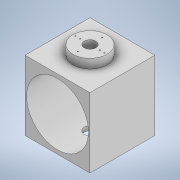
# Autodesk Inventor part: engine_connector_sleeve
Saved by Autodesk Inventor 2020.1 (Build 241239000, 239)
## iProperties
Created: 2022-02-06
Part Number: engine_connector_sleeve
Material: Generic
Document SubType Name: Modeling
Designer: OEM
Density: 1 g/cm^3
Appearance: Default
Author: OEM
Autodesk Inventor part; units mm, degrees
ref_plane "YZ Plane" through (0, 0, 0) normal (1, 0, 0) x (0, 1, 0)
ref_plane "XZ Plane" through (0, 0, 0) normal (0, 1, 0) x (-1, 0, 0)
ref_plane "XY Plane" through (0, 0, 0) normal (0, 0, 1) x (1, 0, 0)
sketch "Sketch1" plane through (0, 0, 0) normal (0, 1, 0) x (-1, 0, 0)
  circle A0 centre (0, 0) radius 11
  circle A1 centre (0, 0) radius 3
  circle A2 centre (0, 0) radius 3.75
  circle A3 centre (0, 0) radius 6.375 construction
  circle A4 centre (0, 0) radius 9.375 construction
  circle A5 centre (0, 0) radius 7.875 construction
  circle A6 centre (0, -7.875) radius 0.35
  circle A7 centre (6.375, 0) radius 0.35
  circle A8 centre (9.375, 0) radius 0.35
  line L0 (16.292, 0) -> (-19, 0) construction
  line L1 (0, 21) -> (0, -27.3544) construction
  circle A9 centre (0, 7.875) radius 0.35
  circle A10 centre (-6.375, 0) radius 0.35
  circle A11 centre (-9.375, 0) radius 0.35
  line L2 (0, -21) -> (21, -21)
  line L3 (21, -21) -> (21, 0)
  line L4 (0, 21) -> (21, 21)
  line L5 (21, 21) -> (21, 0)
  line L6 (0, -21) -> (-21, -21)
  line L7 (-21, -21) -> (-21, 0)
  line L8 (-21, 21) -> (-21, 0)
  line L9 (0, 21) -> (-21, 21)
  dimension "d6" = 12.75
  dimension "d7" = 18.75
  dimension "d8" = 15.75
  dimension "d2" = 7.5
  dimension "d4" = 22
  dimension "d5" = 6
  dimension "d9" = 0.7
  dimension "d13" = 0.7
  dimension "d14" = 0.7
  dimension "d17" = 21
  dimension "d18" = 21
  constraints: 20 end point, 9 centre point, 7 symmetric about line, 6 coincident, 2 horizontal alignment, 1 horizontal, 1 perpendicular, 1 point on line, 1 vertical, 1 vertical alignment, 9 other
  measures "d2" diameter of A2
  measures "d4" diameter of A0
  measures "d5" diameter of A1
  measures "d9" diameter of A6
  measures "d13" diameter of A7
  measures "d14" diameter of A8
  measures "d17" distance from line of point (0, 0) L2
  measures "d18" distance from line of A0.centre L3
extrude "Extrusion1" add sketch "Sketch1" against normal blind 45 contours A0 | A6 | A7 | A8 | A9 | A10 | A11 | L6 L7 L8 L9 L4 L5 L3 L2
extrude "Extrusion2" add sketch "Sketch1" along normal blind 6 contours A0
sketch "Sketch2" plane through (-21, 0, 21) normal (0, 0, 1) x (1, 0, 0)
  line L0 (42, 0) -> (0, 0) construction
  line L1 (42, 0) -> (42, -45) construction
  line L2 (42, -45) -> (0, -45) construction
  line L3 (0, 0) -> (0, -45) construction
  line L4 (42, -45) -> (0, -45) construction
  line L5 (0, 0) -> (0, -45) construction
  line L6 (42, 0) -> (0, -45) construction
  line L7 (42, -45) -> (0, 0) construction
  circle A0 centre (21, -22.5) radius 20
  point P0 (21, 0)
  dimension "d23" = 40
  constraints: 8 end point, 2 perpendicular, 1 centre point, 1 midpoint
  measures "d23" diameter of A0
extrude "Extrusion3" cut sketch "Sketch2" against normal blind 45
equation "\"d13\" = d9"
equation "\"d14\" = d9"
equation "\"d18\" = d17"
body "Solid1"
